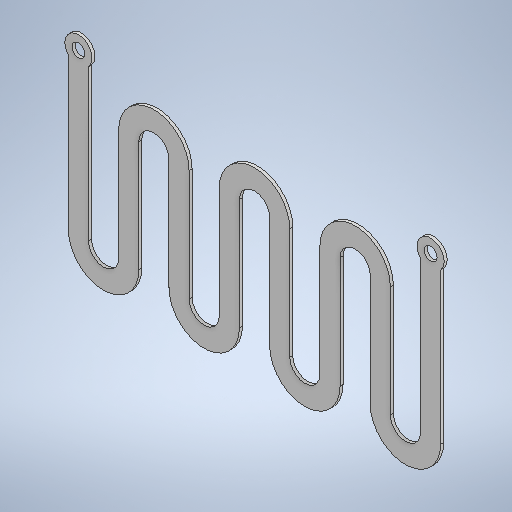
# Autodesk Inventor part: Sensor_0002_001
Saved by Autodesk Inventor 2025.2 (Build 292293000, 293)
## iProperties
Created: 2025-03-20
Part Number: Sensor_0002_001
Material: Genérico
Document SubType Name: Modeling
Designer: lucas
Density: 1 g/cm^3
Appearance: Padrão
Author: lucas
Autodesk Inventor part; units mm, degrees
ref_plane "YZ Plane" through (0, 0, 0) normal (1, 0, 0) x (0, 1, 0)
ref_plane "XZ Plane" through (0, 0, 0) normal (0, 1, 0) x (-1, 0, 0)
ref_plane "XY Plane" through (0, 0, 0) normal (0, 0, 1) x (1, 0, 0)
sketch "Esboço1" plane through (0, 0, 0) normal (0, 0, 1) x (1, 0, 0)
  circle A0 centre (-17500, 10000) radius 1350 construction
  line L0 (-18500, 9093.0821) -> (-18500, -5906.9179)
  line L1 (-16500, 9093.0821) -> (-16500, -5906.9179)
  circle A1 centre (-15000, -5906.9179) radius 1500 construction
  arc A2 (-16500, -5906.9179) -> (-13500, -5906.9179) centre (-15000, -5906.9179) ccw
  circle A3 centre (-15000, -5906.9179) radius 3500 construction
  arc A4 (-18500, -5906.9179) -> (-11500, -5906.9179) centre (-15000, -5906.9179) ccw
  line L2 (-13500, -5906.9179) -> (-13500, 5150)
  line L3 (-11500, -5906.9179) -> (-11500, 5150)
  circle A5 centre (-10000, 5150) radius 1500 construction
  arc A6 (-8500, 5150) -> (-11500, 5150) centre (-10000, 5150) ccw
  circle A7 centre (-10000, 5150) radius 3500 construction
  arc A8 (-6500, 5150) -> (-13500, 5150) centre (-10000, 5150) ccw
  line L4 (-17500, 10000) -> (-17500, 8650) construction
  line L5 (-8500, 5150) -> (-8500, -5906.9179)
  line L6 (-6500, 5150) -> (-6500, -5906.9179)
  circle A9 centre (-5000, -5906.9179) radius 1500 construction
  arc A10 (-6500, -5906.9179) -> (-3500, -5906.9179) centre (-5000, -5906.9179) ccw
  circle A11 centre (-5000, -5906.9179) radius 3500 construction
  arc A12 (-8500, -5906.9179) -> (-1500, -5906.9179) centre (-5000, -5906.9179) ccw
  line L7 (-1500, -5906.9179) -> (-1500, 5150)
  line L8 (6500, 5150) -> (6500, -5906.9179)
  line L9 (1500, -5906.9179) -> (1500, 5150)
  line L10 (3500, -5906.9179) -> (3500, 5150)
  line L11 (-3500, -5906.9179) -> (-3500, 5150)
  line L12 (8500, 5150) -> (8500, -5906.9179)
  circle A13 centre (0, 5150) radius 1500 construction
  circle A14 centre (10000, 5150) radius 1500 construction
  circle A15 centre (5000, -5906.9179) radius 1500 construction
  circle A16 centre (17500, 10000) radius 1350 construction
  circle A17 centre (15000, -5906.9179) radius 1500 construction
  circle A18 centre (0, 5150) radius 3500 construction
  arc A19 (1500, 5150) -> (-1500, 5150) centre (0, 5150) ccw
  arc A20 (3500, 5150) -> (-3500, 5150) centre (0, 5150) ccw
  circle A21 centre (5000, -5906.9179) radius 3500 construction
  arc A22 (3500, -5906.9179) -> (6500, -5906.9179) centre (5000, -5906.9179) ccw
  arc A23 (1500, -5906.9179) -> (8500, -5906.9179) centre (5000, -5906.9179) ccw
  circle A24 centre (10000, 5150) radius 3500 construction
  arc A25 (11500, 5150) -> (8500, 5150) centre (10000, 5150) ccw
  arc A26 (13500, 5150) -> (6500, 5150) centre (10000, 5150) ccw
  line L13 (11500, 5150) -> (11500, -5906.9179)
  line L14 (13500, 5150) -> (13500, -5906.9179)
  line L15 (18500, 9093.0821) -> (18500, -5906.9179)
  line L16 (16500, -5906.9179) -> (16500, 9093.0821)
  circle A27 centre (15000, -5906.9179) radius 3500 construction
  arc A28 (13500, -5906.9179) -> (16500, -5906.9179) centre (15000, -5906.9179) ccw
  arc A29 (11500, -5906.9179) -> (18500, -5906.9179) centre (15000, -5906.9179) ccw
  arc A30 (-16500, 9093.0821) -> (-18500, 9093.0821) centre (-17500, 10000) ccw
  arc A31 (18500, 9093.0821) -> (16500, 9093.0821) centre (17500, 10000) ccw
  circle A32 centre (17500, 10000) radius 650
  circle A33 centre (-17500, 10000) radius 650
  circle A34 centre (-4850, -54944) radius 1350 construction
  line L17 (-3943.0821, -55944) -> (11056.9179, -55944)
  line L18 (-3943.0821, -53944) -> (11056.9178, -53944)
  circle A35 centre (11056.9179, -52444) radius 1500 construction
  arc A36 (11056.9178, -53944) -> (11056.9179, -50944) centre (11056.9178, -52444) ccw
  circle A37 centre (11056.9179, -52444) radius 3500 construction
  arc A38 (11056.9179, -55944) -> (11056.9179, -48944) centre (11056.9179, -52444) ccw
  line L19 (11056.9179, -50944) -> (2.8909, -50943.9988)
  line L20 (11056.9179, -48944) -> (0, -48944)
  circle A39 centre (0, -47444) radius 1500 construction
  arc A40 (0, -45944) -> (0, -48944) centre (0, -47444) ccw
  circle A41 centre (0, -47444) radius 3500 construction
  arc A42 (0, -43944) -> (2.8909, -50943.9988) centre (0, -47444) ccw
  line L21 (-4850, -54944) -> (-3500, -54944) construction
  line L22 (0, -45944) -> (11056.9179, -45944)
  line L23 (0, -43944) -> (11056.9179, -43944)
  circle A43 centre (11056.9179, -42444) radius 1500 construction
  arc A44 (11056.9179, -43944) -> (11056.9179, -40944) centre (11056.9179, -42444) ccw
  circle A45 centre (11056.9179, -42444) radius 3500 construction
  arc A46 (11056.9179, -45944) -> (11056.9179, -38944) centre (11056.9179, -42444) ccw
  line L24 (11056.9179, -38944) -> (0, -38944)
  line L25 (0, -30944) -> (11056.9179, -30944)
  line L26 (11056.9179, -35944) -> (0, -35944)
  line L27 (11056.9179, -33944) -> (0, -33944)
  line L28 (11056.9179, -40944) -> (0, -40944)
  line L29 (0, -28944) -> (11056.9179, -28944)
  circle A47 centre (0, -37444) radius 1500 construction
  circle A48 centre (0, -27444) radius 1500 construction
  circle A49 centre (11056.9179, -32444) radius 1500 construction
  circle A50 centre (-4850, -19944) radius 1350 construction
  circle A51 centre (11056.9179, -22444) radius 1500 construction
  circle A52 centre (0, -37444) radius 3500 construction
  arc A53 (0, -35944) -> (0, -38944) centre (0, -37444) ccw
  arc A54 (0, -33944) -> (0, -40944) centre (0, -37444) ccw
  circle A55 centre (11056.9179, -32444) radius 3500 construction
  arc A56 (11056.9179, -33944) -> (11056.9179, -30944) centre (11056.9179, -32444) ccw
  arc A57 (11056.9179, -35944) -> (11056.9179, -28944) centre (11056.9179, -32444) ccw
  circle A58 centre (0, -27444) radius 3500 construction
  arc A59 (0, -25944) -> (0, -28944) centre (0, -27444) ccw
  arc A60 (0, -23944) -> (0, -30944) centre (0, -27444) ccw
  line L30 (0, -25944) -> (11056.9179, -25944)
  line L31 (0, -23944) -> (11056.9179, -23944)
  line L32 (-3943.0821, -18944) -> (11056.9179, -18944)
  line L33 (11056.9179, -20944) -> (-3943.0821, -20944)
  circle A61 centre (11056.9179, -22444) radius 3500 construction
  arc A62 (11056.9179, -23944) -> (11056.9179, -20944) centre (11056.9179, -22444) ccw
  arc A63 (11056.9179, -25944) -> (11056.9179, -18944) centre (11056.9179, -22444) ccw
  arc A64 (-3943.0821, -53944) -> (-3943.0821, -55944) centre (-4850, -54944) ccw
  arc A65 (-3943.0821, -18944) -> (-3943.0821, -20944) centre (-4850, -19944) ccw
  circle A66 centre (-4850, -19944) radius 650
  circle A67 centre (-4850, -54944) radius 650
  point P0 (0, 0)
  point P1 (-15000, -7406.9179)
  point P2 (-10000, 8650)
  point P3 (0, 6650)
  point P4 (0, 8650)
  point P5 (15000, -7406.9179)
  point P6 (3500, -5906.9179)
  point P7 (12556.9178, -52444)
  point P8 (-3499.9997, -47445.4454)
  point P9 (-1500, -37444)
  point P10 (-3500, -37444)
  point P11 (12556.9179, -22444)
  dimension "d7" = 3000
  dimension "d0" = 10000
  dimension "d1" = 17500
  dimension "d2" = 2700
  dimension "d5" = 15000
  dimension "d8" = 2000
  dimension "d12" = 1300
  constraints: 108 point on circle, 68 end point, 52 centre point, 34 horizontal alignment, 22 vertical, 13 parallel, 13 tangent, 10 vertical alignment, 9 concentric, 2 coincident, 2 point on line, 1 equal radius, 49 other
  measures "d0" vertical distance of point (0, 0) L4.start
  measures "d1" horizontal distance of point (0, 0) L4.start
  measures "d2" diameter of A0
  measures "d5" distance of L1.start L1.end
  measures "d8" distance between parallel lines of L1 L0
  measures "d12" diameter of A33
extrude "Extrusão1" add sketch "Esboço1" along normal mid plane 300 contours A30 L1 A2 L2 A8 L6 A10 L11 A20 L10 A22 L8 A26 L14 A28 L16 A31 L15 A29 L13 A25 L12 A23 L9 A19 L7 A12 L5 A6 L3 A4 L0
